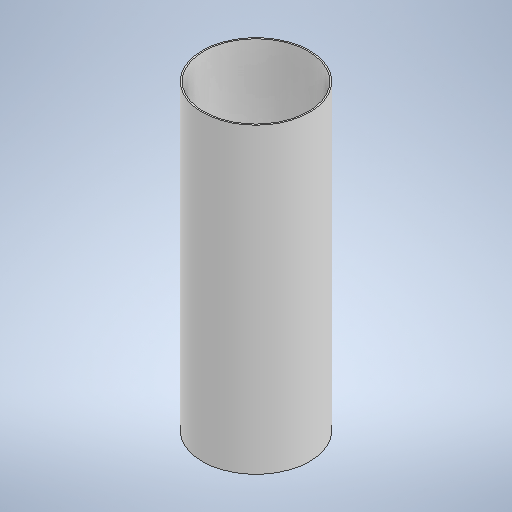
# Autodesk Inventor part: 1
Saved by Autodesk Inventor 2025 (Build 290162000, 162)
## iProperties
Created: 2024-07-23
Part Number: 1
Material: Generic
Document SubType Name: Modeling
Designer: User
Density: 1 g/cm^3
Appearance: Default
Author: User
Autodesk Inventor part; units mm, degrees
ref_plane "YZ Plane" through (0, 0, 0) normal (1, 0, 0) x (0, 1, 0)
ref_plane "XZ Plane" through (0, 0, 0) normal (0, 1, 0) x (-1, 0, 0)
ref_plane "XY Plane" through (0, 0, 0) normal (0, 0, 1) x (1, 0, 0)
sketch "Sketch1" plane through (0, 0, 0) normal (0, 0, 1) x (1, 0, 0)
  line L0 (-10, 0) -> (-38, 0)
  line L1 (-38, 0) -> (-38, 60)
  arc A0 (0, 10) -> (-10, 0) centre (0, 0) ccw
  line L2 (0, 10) -> (0, 100)
  line L3 (0, 100) -> (-15, 100)
  line L4 (-15, 100) -> (-15, 80)
  line L5 (0, 10) -> (0, 0)
  line L6 (-38, 60) -> (-15, 80)
  dimension "d5" = 60
  dimension "d9" = 20
  dimension "d11" = 15
  dimension "d12" = 20
  constraints: 14 end point, 4 vertical, 2 point on circle, 1 centre point, 1 horizontal, 1 perpendicular
  measures "d5" distance of L0.end L1.end
  measures "d9" diameter of A0
  measures "d11" distance of L2.end L3.end
  measures "d12" distance of L3.end L4.end
revolve "Revolution1" add sketch "Sketch1" angle 360 about axis through (0, 10, 0) along (0, 1, 0)
fillet "Fillet1" radius 10 1 edges at (15, 80, 0)
fillet "Fillet1" radius 20 1 edges at (38, 60, 0)
fillet "Fillet3" radius 10 1 edges at (10, 0, 0)
shell "Shell1" thickness 1 removed faces 1 at (4.4273, 100, -2.3236)
sketch "Sketch2" plane through (0, 0, 0) normal (1, 0, 0) x (0, 1, 0)
  line L0 (100, -15) -> (100, 15) projected
  line L1 (100, 0) -> (90, 0)
  circle A0 centre (90, 0) radius 3.5
  point P0 (0, 0)
  dimension "d20" = 10
  dimension "d21" = 7
  constraints: 2 end point, 1 centre point, 1 coincident, 1 horizontal, 1 midpoint
  measures "d20" distance of L1.start L1.end
  measures "d21" diameter of A0
extrude "Extrusion1" cut sketch "Sketch2" along normal mid plane 50
sketch "Sketch3" plane through (0, 0, 0) normal (0, -1, 0) x (1, 0, 0)
  circle A0 centre (0, 0) radius 37 projected
  circle A1 centre (0, 0) radius 38
  circle A2 centre (0, 0) radius 39
  dimension "d24" = 76
  dimension "d25" = 78
  constraints: 2 centre point, 2 coincident
  measures "d24" diameter of A1
  measures "d25" diameter of A2
extrude "Extrusion2" add sketch "Sketch3" against normal blind 220 contours A2
body "Solid1"
